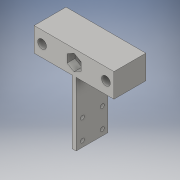
# Autodesk Inventor part: Traveller
Saved by Autodesk Inventor 2016 (Build 200138000, 138)
## iProperties
Created: 2016-04-14
Part Number: Traveller
Material: Generic
Document SubType Name: Modeling
Designer: rmarkowi
Density: 1 g/cm^3
Appearance: Default
Author: rmarkowi
Autodesk Inventor part; units mm, degrees
ref_plane "YZ Plane" through (0, 0, 0) normal (1, 0, 0) x (0, 1, 0)
ref_plane "XZ Plane" through (0, 0, 0) normal (0, 1, 0) x (-1, 0, 0)
ref_plane "XY Plane" through (0, 0, 0) normal (0, 0, 1) x (1, 0, 0)
sketch "Sketch1" plane through (0, 0, 0) normal (0, 1, 0) x (-1, 0, 0)
  line L0 (0, 0) -> (127, 0)
  line L1 (127, 0) -> (127, -50.8)
  line L2 (127, -50.8) -> (0, -50.8)
  line L3 (0, -50.8) -> (0, 0)
  dimension "d0" = 127
  dimension "d1" = 50.8
  constraints: 8 end point, 2 parallel, 1 horizontal, 1 perpendicular
  measures "d0" distance of L1.end L2.end
  measures "d1" distance of L0.end L1.end
extrude "Extrusion1" add sketch "Sketch1" along normal blind 38.1
sketch "Sketch2" plane through (-127, 0, 0) normal (0, 0, 1) x (1, 0, 0)
  line L0 (123.825, 0) -> (3.175, 0) construction
  circle A0 centre (63.4683, 18.9303) radius 6.985
  circle A1 centre (12.6683, 18.9303) radius 6.985
  circle A2 centre (114.2683, 18.9303) radius 6.985
  line L1 (63.5, 0) -> (63.5, 25.2805) construction
  line L2 (127, 0) -> (127, 38.1) construction
  line L3 (127, 19.05) -> (0, 19.05) construction
  point P0 (0, -12.7)
  dimension "d4" = 13.97
  dimension "d5" = 13.97
  dimension "d8" = 13.97
  dimension "d9" = 50.8
  dimension "d10" = 50.8
  constraints: 6 end point, 3 centre point, 2 midpoint, 1 horizontal
  measures "d4" diameter of A0
  measures "d5" diameter of A1
  measures "d8" diameter of A2
  measures "d9" distance of A1.centre A0.centre
  measures "d10" distance of A2.centre A0.centre
extrude "Extrusion2" cut sketch "Sketch2" against normal through all
sketch "Sketch3" plane through (-127, 0, 0) normal (0, 0, 1) x (1, 0, 0)
  circle A0 centre (63.4683, 18.9303) radius 6.985 projected
  line L0 (63.4683, 31.7619) -> (74.5808, 25.3461)
  line L1 (74.5808, 25.3461) -> (74.5808, 12.5145)
  line L2 (74.5808, 12.5145) -> (63.4683, 6.0987)
  line L3 (63.4683, 6.0987) -> (52.3558, 12.5145)
  line L4 (52.3558, 12.5145) -> (52.3558, 25.3461)
  line L5 (52.3558, 25.3461) -> (63.4683, 31.7619)
  point P0 (127, 0)
  dimension "d11" = 22.225
  constraints: 12 end point, 1 coincident, 13 other
  measures "d11" distance between parallel lines of L4 L1
extrude "Extrusion3" cut sketch "Sketch3" against normal blind 12.7
sketch "Sketch4" plane through (0, 0, -50.8) normal (0, 0, -1) x (-1, 0, 0)
  line L0 (63.4683, 31.7619) -> (74.5808, 25.3461)
  line L1 (74.5808, 25.3461) -> (74.5808, 12.5145)
  line L2 (74.5808, 12.5145) -> (63.4683, 6.0987)
  line L3 (63.4683, 6.0987) -> (52.3558, 12.5145)
  line L4 (52.3558, 12.5145) -> (52.3558, 25.3461)
  line L5 (52.3558, 25.3461) -> (63.4683, 31.7619)
  point P0 (0, 0)
  point P1 (127, 0)
  point P2 (63.4683, 18.9303)
  dimension "d14" = 22.225
  constraints: 12 end point, 13 other
  measures "d14" distance between parallel lines of L4 L1
extrude "Extrusion5" cut sketch "Sketch4" against normal blind 12.7
sketch "Sketch5" plane through (0, 0, 0) normal (0, -1, 0) x (1, 0, 0)
  line L0 (-63.4683, -50.8) -> (-66.6433, -50.8)
  line L1 (-66.6433, -50.8) -> (-66.6433, 0)
  line L2 (-66.6433, 0) -> (-63.4683, 0)
  line L3 (-63.4683, 0) -> (-63.4683, -50.8) construction
  line L4 (-63.4683, -50.8) -> (-60.2933, -50.8)
  line L5 (-60.2933, -50.8) -> (-60.2933, 0)
  line L6 (-60.2933, 0) -> (-63.4683, 0)
  point P0 (0, 0)
  dimension "d19" = 3.175
  dimension "d20" = 50.8
  constraints: 14 end point, 2 parallel, 2 symmetric about line, 1 horizontal, 1 perpendicular
  measures "d19" distance of L1.end L2.end
  measures "d20" distance of L0.end L1.end
extrude "Extrusion6" add sketch "Sketch5" along normal blind 101.6
sketch "Sketch6" plane through (-66.6433, 0, -50.8) normal (-1, 0, 0) x (0, 0, 1)
  line L0 (0, 0) -> (0, -101.6) construction
  line L1 (0, -101.6) -> (50.8, -101.6) construction
  line L2 (50.8, -101.6) -> (50.8, -50.8) construction
  line L3 (50.8, -50.8) -> (0, -50.8) construction
  line L4 (0, -50.8) -> (0, -101.6) construction
  line L5 (0, -50.8) -> (49.9098, -101.6) construction
  line L6 (9.0799, -92.075) -> (40.8299, -92.075) construction
  line L7 (40.8299, -92.075) -> (40.8299, -60.325) construction
  line L8 (40.8299, -60.325) -> (9.0799, -60.325) construction
  line L9 (9.0799, -60.325) -> (9.0799, -92.075) construction
  line L10 (9.0799, -92.075) -> (40.8299, -60.325) construction
  line L11 (40.8299, -92.075) -> (9.0799, -60.325) construction
  circle A0 centre (40.8299, -60.325) radius 3.175
  circle A1 centre (40.8299, -92.075) radius 3.175
  circle A2 centre (9.0799, -92.075) radius 3.175
  circle A3 centre (9.0799, -60.325) radius 3.175
  point P0 (50.8, 0)
  point P1 (24.9549, -76.2)
  dimension "d23" = 50.8
  dimension "d24" = 50.8
  dimension "d25" = 31.75
  dimension "d26" = 31.75
  dimension "d27" = 6.35
  dimension "d28" = 6.35
  dimension "d29" = 6.35
  dimension "d30" = 6.35
  constraints: 22 end point, 4 centre point, 4 parallel, 3 midpoint, 2 horizontal, 2 perpendicular, 1 coincident, 1 point on line
  measures "d23" distance of L3.end L2.end
  measures "d24" distance of L2.end L1.end
  measures "d25" distance of L8.end L7.end
  measures "d26" distance of L7.end L6.end
  measures "d27" diameter of A0
  measures "d28" diameter of A1
  measures "d29" diameter of A2
  measures "d30" diameter of A3
extrude "Extrusion7" cut sketch "Sketch6" against normal through all
body "Solid1"
